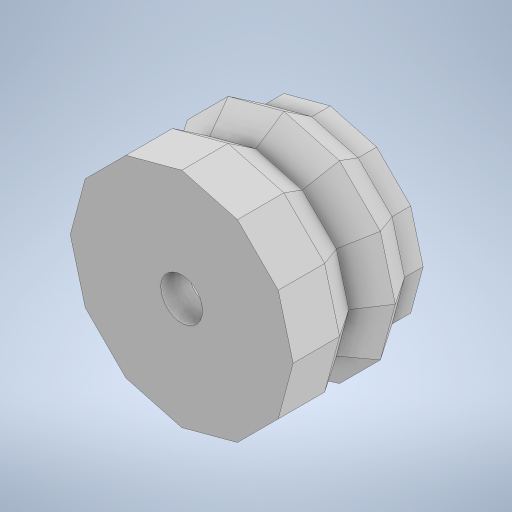
# Autodesk Inventor part: Test6
Saved by Autodesk Inventor 2023 (Build 270158000, 158)
## iProperties
Created: 2024-07-03
Part Number: Test6
Material: 일반
Document SubType Name: Modeling
Designer: ojs08
Density: 1 g/cm^3
Appearance: 기본값
Author: ojs08
Autodesk Inventor part; units mm, degrees
ref_plane "YZ Plane" through (0, 0, 0) normal (1, 0, 0) x (0, 1, 0)
ref_plane "XZ Plane" through (0, 0, 0) normal (0, 1, 0) x (-1, 0, 0)
sketch "스케치1" plane through (0, 0, 0) normal (0, 0, 1) x (1, 0, 0)
  line L0 (10.392305, 6) -> (12, 0)
  line L1 (12, 0) -> (10.392305, -6)
  line L2 (10.392305, -6) -> (6, -10.392305)
  line L3 (6, -10.392305) -> (0, -12)
  line L4 (0, -12) -> (-6, -10.392305)
  line L5 (-6, -10.392305) -> (-10.392305, -6)
  line L6 (-10.392305, -6) -> (-12, 0)
  line L7 (-12, 0) -> (-10.392305, 6)
  line L8 (-10.392305, 6) -> (-6, 10.392305)
  line L9 (-6, 10.392305) -> (0, 12)
  line L10 (0, 12) -> (6, 10.392305)
  line L11 (6, 10.392305) -> (10.392305, 6)
  line L12 (-16.8, 0) -> (16.8, 0)
  point P0 (0, 0)
  point P1 (0, 0)
  dimension "d0" = 24
  constraints: 24 end point, 1 coincident, 1 point on line, 25 other
  measures "d0" distance of L0.end L6.end
ref_plane "작업 평면1" through (0, 0, 3) normal (0, 0, 1) x (1, 0, 0)
sketch "스케치2" plane through (0, 0, 3) normal (0, 0, 1) x (1, 0, 0)
  line L0 (10, 0) -> (8.660254, -5)
  line L1 (8.660254, -5) -> (5, -8.660254)
  line L2 (5, -8.660254) -> (0, -10)
  line L3 (0, -10) -> (-5, -8.660254)
  line L4 (-5, -8.660254) -> (-8.660254, -5)
  line L5 (-8.660254, -5) -> (-10, 0)
  line L6 (-10, 0) -> (-8.660254, 5)
  line L7 (-8.660254, 5) -> (-5, 8.660254)
  line L8 (-5, 8.660254) -> (0, 10)
  line L9 (0, 10) -> (5, 8.660254)
  line L10 (5, 8.660254) -> (8.660254, 5)
  line L11 (8.660254, 5) -> (10, 0)
  line L12 (-16.8, 0) -> (16.8, 0)
  point P0 (0, 0)
  point P1 (0, 0)
  dimension "d2" = 20
  constraints: 24 end point, 1 coincident, 1 point on line, 25 other
  measures "d2" distance of L0.start L5.end
loft "로프트1" add profiles "스케치1", "스케치2"
mirror "미러1" about plane through (0, 0, 3) normal (0, 0, 1) of "로프트1"
mirror "미러2" about plane through (0, 0, 0) normal (0, 0, -1) of "로프트1"
sketch "스케치3" plane through (12, 0, 6) normal (0, 0, 1) x (0.9659258, 0.258819, 0)
  line L0 (0, 6.211657) -> (0, 0)
  line L1 (-3.105829, 11.59111) -> (0, 6.211657)
  line L2 (-8.485281, 14.696938) -> (-3.105829, 11.59111)
  line L3 (-14.696938, 14.696938) -> (-8.485281, 14.696938)
  line L4 (-20.076391, 11.59111) -> (-14.696938, 14.696938)
  line L5 (-23.18222, 6.211657) -> (-20.076391, 11.59111)
  line L6 (-23.18222, 0) -> (-23.18222, 6.211657)
  line L7 (-20.076391, -5.379453) -> (-23.18222, 0)
  line L8 (-14.696938, -8.485281) -> (-20.076391, -5.379453)
  line L9 (-8.485281, -8.485281) -> (-14.696938, -8.485281)
  line L10 (-3.105829, -5.379453) -> (-8.485281, -8.485281)
  line L11 (0, 0) -> (-3.105829, -5.379453)
  point P0 (-11.59111, 3.105829)
extrude "돌출1" add sketch "스케치3" along normal blind 2.5
shell "쉘1" thickness 0.5 removed faces 0 ; own thickness 2 on faces at (7.049429, 8.432192, -1) (10.321081, 3.777778, -1) (10.827207, -1.888889, -1) (8.432192, -7.049429, -1) (3.777778, -10.321081, -1) (-1.888889, -10.827207, -1) (-7.049429, -8.432192, -1) (-10.321081, -3.777778, -1) (-10.827207, 1.888889, -1) (-8.432192, 7.049429, -1) (-3.777778, 10.321081, -1) (1.888889, 10.827207, -1) (-3.777778, 10.321081, 5) (1.888889, 10.827207, 5) (-8.432192, 7.049429, 5) (-10.827207, 1.888889, 5) (-10.321081, -3.777778, 5) (-7.049429, -8.432192, 5) (-1.888889, -10.827207, 5) (3.777778, -10.321081, 5) (8.432192, -7.049429, 5) (10.321081, 3.777778, 5) (10.827207, -1.888889, 5) (7.049429, 8.432192, 5)
sketch "스케치4" plane through (12, 0, 8.5) normal (0, 0, 1) x (0.9659258, 0.258819, 0)
  line L0 (-3.105829, 11.59111) -> (-8.485281, 14.696938)
  line L1 (-8.485281, 14.696938) -> (-14.696938, 14.696938)
  line L2 (-14.696938, 14.696938) -> (-20.076391, 11.59111)
  line L3 (-20.076391, 11.59111) -> (-23.18222, 6.211657)
  line L4 (-23.18222, 6.211657) -> (-23.18222, 0)
  line L5 (-23.18222, 0) -> (-20.076391, -5.379453)
  line L6 (-20.076391, -5.379453) -> (-14.696938, -8.485281)
  line L7 (-14.696938, -8.485281) -> (-8.485281, -8.485281)
  line L8 (-8.485281, -8.485281) -> (-3.105829, -5.379453)
  line L9 (-3.105829, -5.379453) -> (0, 0)
  line L10 (0, 0) -> (0, 6.211657)
  line L11 (0, 6.211657) -> (-3.105829, 11.59111)
  point P0 (-11.59111, 3.105829)
extrude "돌출2" add sketch "스케치4" along normal blind 2.5
sketch "스케치5" plane through (12, 0, 11) normal (0, 0, 1) x (0.9659258, 0.258819, 0)
  circle A0 centre (-11.59111, 3.105829) radius 2.25
  dimension "d13" = 4.5
  constraints: 1 centre point, 1 coincident
  measures "d13" diameter of A0
extrude "돌출3" cut sketch "스케치5" against normal blind 3
sketch "스케치6" plane through (10, 0, -3) normal (0, 0, -1) x (-0.9659258, -0.258819, 0)
  line L0 (0, 5.176381) -> (0, 0)
  line L1 (0, 0) -> (2.58819, -4.482877)
  line L2 (2.58819, -4.482877) -> (7.071068, -7.071068)
  line L3 (7.071068, -7.071068) -> (12.247449, -7.071068)
  line L4 (12.247449, -7.071068) -> (16.730326, -4.482877)
  line L5 (16.730326, -4.482877) -> (19.318517, 0)
  line L6 (19.318517, 0) -> (19.318517, 5.176381)
  line L7 (19.318517, 5.176381) -> (16.730326, 9.659258)
  line L8 (16.730326, 9.659258) -> (12.247449, 12.247449)
  line L9 (12.247449, 12.247449) -> (7.071068, 12.247449)
  line L10 (7.071068, 12.247449) -> (2.58819, 9.659258)
  line L11 (2.58819, 9.659258) -> (0, 5.176381)
  point P0 (9.659258, 2.58819)
extrude "돌출4" add sketch "스케치6" along normal blind 2
